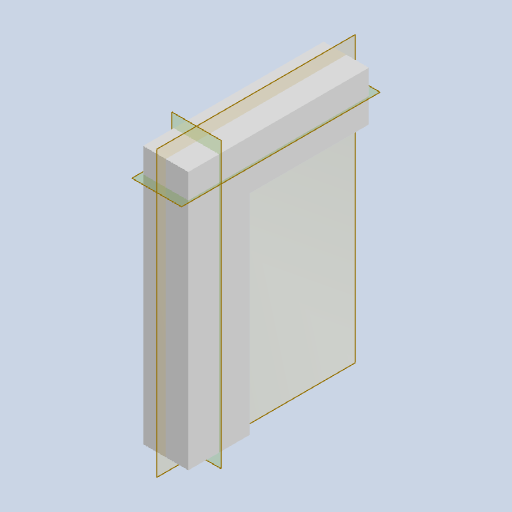
# Autodesk Inventor part: Head Posts
Saved by Autodesk Inventor 2022 (Build 260153000, 153)
## iProperties
Created: 2022-01-18
Part Number: Head Posts
Material: Generic
Document SubType Name: Modeling
Designer: gnzak
Density: 1 g/cm^3
Appearance: Default
Author: gnzak
Autodesk Inventor part; units mm, degrees
ref_plane "YZ Plane" through (0, 0, 0) normal (1, 0, 0) x (0, 1, 0)
ref_plane "XZ Plane" through (0, 0, 0) normal (0, 1, 0) x (-1, 0, 0)
ref_plane "XY Plane" through (0, 0, 0) normal (0, 0, 1) x (1, 0, 0)
sketch "Sketch1" plane through (0, 0, 0) normal (1, 0, 0) x (0, 1, 0)
  line L0 (29.4716, 1.335) -> (29.4716, -68.515)
  line L1 (29.4716, -68.515) -> (10.4216, -68.515)
  line L2 (10.4216, -68.515) -> (10.4216, -22.4775)
  line L3 (10.4216, -22.4775) -> (-70.5409, -22.4775)
  line L4 (-70.5409, -22.4775) -> (-70.5409, 1.335)
  line L5 (-70.5409, 1.335) -> (29.4716, 1.335)
  point P0 (0, 0)
  dimension "d0" = 69.85
  dimension "d1" = 46.0375
  dimension "d2" = 23.8125
  dimension "d3" = 100.0125
  dimension "d4" = 19.05
  constraints: 12 end point, 4 perpendicular, 1 vertical
  measures "d0" distance of L0.start L0.end
  measures "d1" distance of L1.end L2.end
  measures "d2" distance of L3.end L4.end
  measures "d3" distance of L4.end L0.start
  measures "d4" distance of L0.end L1.end
extrude "Extrusion1" add sketch "Sketch1" along normal blind 17.4625
ref_plane "Work Plane1" through (0, -70.5409, -10.5712) normal (0, 0, -1) x (-1, 0, 0)
ref_plane "Work Plane2" through (8.7313, 0, 0) normal (1, 0, 0) x (0, 0, -1)
ref_plane "Work Plane3" through (0, 19.9466, -68.515) normal (0, -1, 0) x (1, 0, 0)
equation "\"d1\" = d0 - d2"
body "Solid1"
